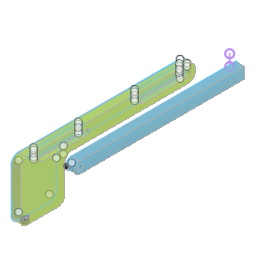
AA_Extended (Autodesk Fusion 360 design; units mm, degrees)
Autodesk Fusion 360 part; units mm, degrees
sketch "Sketch1" plane through (0, 0, 0) normal (1, 0, 0) x (0, 1, 0) in component "Arm"
  line L0 (239.539, 35.8777) -> (53.0265, 35.8777)
  line L1 (239.539, 23.1777) -> (239.539, 35.8777)
  line L2 (239.539, 23.1777) -> (53.0265, 23.1777)
  circle A0 centre (53.0265, 29.5277) radius 3.175
  arc A1 (53.0265, 35.8777) -> (53.0265, 23.1777) centre (53.0265, 29.5277) ccw
  point P0 (46.6765, 29.5277)
  dimension "d23" = 12.7
  dimension "d24" = 6.35
  dimension "d25" = 6.35
  dimension "d26" = 192.8625
  constraint concentric A0 A1
  constraint parallel L0 L2
  constraint midpoint A1 P0
  measures "d23" distance of L0 L2
  measures "d24" diameter of A0
  measures "d25" radius of A1
  measures "d26" distance of L1 P0
extrude "Extrude2" add sketch "Sketch1" along normal blind 9.525 makes body 1 in component "Arm"
sketch "Sketch1 (2)" plane through (0, 0, 0) normal (1, 0, 0) x (0, 1, 0) in component "BasePlate"
  line L0 (34.929, -7.9375) -> (0, -7.9375)
  line L1 (42.8665, 31.7502) -> (42.8665, 0)
  arc A0 (50.804, 39.6877) -> (42.8665, 31.7502) centre (50.804, 31.7502) ccw
  line L2 (183.1472, 39.6877) -> (50.804, 39.6877)
  arc A1 (183.1472, 39.6877) -> (191.0847, 47.6252) centre (183.1472, 47.6252) ccw
  line L3 (191.0847, 50.8002) -> (191.0847, 47.6252)
  arc A2 (191.0847, 50.8002) -> (183.1472, 58.7377) centre (183.1472, 50.8002) ccw
  line L4 (0, 58.7377) -> (183.1472, 58.7377)
  line L5 (-7.9375, 0) -> (-7.9375, 50.8002)
  circle A3 centre (0, 0) radius 2.54
  line L6 (16.9677, 43.6247) -> (67.7677, 43.6247)
  arc A4 (16.9677, 54.8007) -> (16.9677, 43.6247) centre (16.9677, 49.2127) ccw
  arc A5 (16.9677, 52.4512) -> (16.9677, 45.9742) centre (16.9677, 49.2127) ccw
  line L7 (16.9677, 52.4512) -> (67.7677, 52.4512)
  line L8 (67.7677, 45.9742) -> (16.9677, 45.9742)
  arc A6 (67.7677, 45.9742) -> (67.7677, 52.4512) centre (67.7677, 49.2127) ccw
  line L9 (67.7677, 54.8007) -> (16.9677, 54.8007)
  arc A7 (67.7677, 43.6247) -> (67.7677, 54.8007) centre (67.7677, 49.2127) ccw
  arc A8 (131.5217, 54.8007) -> (131.5217, 43.6247) centre (131.5217, 49.2127) ccw
  line L10 (131.5217, 43.6247) -> (182.3217, 43.6247)
  arc A9 (182.3217, 43.6247) -> (182.3217, 54.8007) centre (182.3217, 49.2127) ccw
  arc A10 (182.3217, 45.9742) -> (182.3217, 52.4512) centre (182.3217, 49.2127) ccw
  line L11 (131.5217, 52.4512) -> (182.3217, 52.4512)
  line L12 (182.3217, 54.8007) -> (131.5217, 54.8007)
  arc A11 (131.5217, 52.4512) -> (131.5217, 45.9742) centre (131.5217, 49.2127) ccw
  line L13 (182.3217, 45.9742) -> (131.5217, 45.9742)
  arc A12 (0, 58.7377) -> (-7.9375, 50.8002) centre (0, 50.8002) ccw
  arc A13 (-7.9375, 0) -> (0, -7.9375) centre (0, 0) ccw
  arc A14 (34.929, -7.9375) -> (42.8665, 0) centre (34.929, 0) ccw
  line L14 (239.539, 23.1777) -> (239.539, 35.8777)
  dimension "d17" = 66.6752
  dimension "d18" = 50.804
  dimension "d19" = 7.9375
  dimension "d20" = 19.05
  dimension "d21" = 199.0222
  dimension "d27" = 50.8
  dimension "d28" = 50.8
  dimension "d29" = 6.477
  dimension "d30" = 11.176
  dimension "d31" = 5.08
  constraint tangent L5 A12
  constraint tangent L4 A12
  constraint tangent L5 A13
  constraint tangent L0 A13
  constraint equal A12 A13
  constraint tangent L0 A14
  constraint tangent L1 A14
  constraint equal A12 A14
  measures "d17" distance of L0 L4
  measures "d18" distance of L1 L5
  measures "d19" radius of A12
  measures "d20" distance of L2 L4
  measures "d21" distance of L3 L5
  measures "d27" distance of A4.centre A6.centre
  measures "d28" distance of A8.centre A9.centre
  measures "d29" distance of L7 L8
  measures "d30" distance of L6 L9
  measures "d31" diameter of A3
extrude "Extrude3" add sketch "Sketch1 (2)" along normal blind 9.525 separate body contours L0 L1 A0 L2 A1 L3 A2 L4 L5 A12 A13 A14 | L6 A4 L9 A7 | A8 L10 A9 L12 makes body 2 in component "Arm"
extrude "Extrude4" cut sketch "Sketch1 (2)" along normal blind 4.445 contours L6 A4 L9 A7 | A8 L10 A9 L12 bodies 2 in component "Arm"
thread "Thread1" "ANSI Unified Screw Threads 0.25 1/4-20 UNC 3B" major diameter 6.35 minor diameter 5.1156 pitch 1.27 angle 60 resizes the face on face at (6.35, 2.5368, -0.1266) on bodies 2 in component "Arm"
copy_body "CutPasteBodies1" bodies 2 removing the originals makes body 3 in component "BasePlate"
thread "Thread1'" "ANSI Unified Screw Threads 0.25 1/4-20 UNC 3B" major diameter 6.35 minor diameter 5.1156 pitch 1.27 angle 60 resizes the face on face at (3.175, 2.5546, 0.1275) on bodies 3 in component "BasePlate"
component "Arm" placed x (1, 0, 0) y (0, 1, 0) z (0, 0, 1) at (0, 7.0889, -11.1651)
component "BasePlate" placed x (1, 0, 0) y (0, 1, 0) z (0, 0, 1) at (0, 0, 0)
equation "d159_1 = 0.00000 in"
equation "d160_1 = 0.0000 deg"
